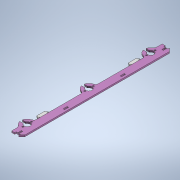
# Autodesk Inventor part: chassis_1_1-02
Saved by Autodesk Inventor 2022 (Build 260153000, 153)
## iProperties
Created: 2023-03-24
Part Number: chassis_1_1-02
Material: 一般
Document SubType Name: Modeling
Designer: Johnny Jou
Density: 1 g/cm^3
Appearance: 預設
Author: Johnny Jou
Autodesk Inventor part; units mm, degrees
ref_plane "YZ Plane" through (0, 0, 0) normal (1, 0, 0) x (0, 1, 0)
ref_plane "XZ Plane" through (0, 0, 0) normal (0, 1, 0) x (-1, 0, 0)
ref_plane "XY Plane" through (0, 0, 0) normal (0, 0, 1) x (1, 0, 0)
sketch "草圖1" plane through (0, 0, 0) normal (0, 1, 0) x (-1, 0, 0)
  line L0 (0, 0) -> (0, -296)
  arc A0 (15, -160.4599) -> (15, -135.5401) centre (16, -148) ccw
  circle A1 centre (16, -148) radius 26 construction
  line L1 (15, -286) -> (15, -160.4599)
  line L2 (15, -135.5401) -> (15, -10)
  circle A2 centre (16, -139.5) radius 1.5
  circle A3 centre (16, -156.5) radius 1.5
  line L3 (20, 0) -> (20, -10)
  line L4 (20, -10) -> (15, -10)
  line L5 (0, -10) -> (0, 0)
  line L6 (6, 0) -> (6, -3)
  line L7 (6, -3) -> (14, -3)
  line L8 (14, -3) -> (14, 0)
  line L9 (0, 0) -> (6, 0)
  line L10 (14, 0) -> (20, 0)
  line L11 (15, 0) -> (14, 0)
  line L12 (6, 0) -> (0, 0)
  line L13 (20, -296) -> (20, -286)
  line L14 (20, -286) -> (15, -286)
  line L15 (0, -290) -> (0, -296)
  line L16 (6, -296) -> (6, -293)
  line L17 (6, -293) -> (14, -293)
  line L18 (14, -293) -> (14, -296)
  line L19 (0, -296) -> (6, -296)
  line L20 (14, -296) -> (20, -296)
  dimension "d1" = 15
  dimension "d2" = 25
  dimension "d3" = 52
  dimension "d4" = 16
  dimension "d6" = 3
  dimension "d7" = 17
  dimension "d8" = 8.5
  dimension "d9" = 10
  dimension "d10" = 20
  dimension "d11" = 8
  dimension "d12" = 3
  dimension "d13" = 6
  dimension "d15" = 3
  dimension "d16" = 8
  dimension "d17" = 6
  dimension "d34" = 296
  dimension "d35" = 148
  dimension "d36" = 10
  dimension "d55" = 8.5
  dimension "d56" = 15
  dimension "d57" = 15
  constraints: 42 end point, 10 parallel, 6 horizontal, 6 perpendicular, 4 centre point, 2 coincident, 2 collinear, 2 point on circle, 1 equal radius, 1 vertical alignment
  measures "d1" distance of L11.start L0.start
  measures "d2" diameter of A0
  measures "d3" diameter of A1
  measures "d4" distance from line of L0 A0.centre
  measures "d6" diameter of A2
  measures "d7" distance of A3.centre A2.centre
  measures "d8" distance of A0.centre A3.centre
  measures "d9" distance of L3.start L3.end
  measures "d10" distance between parallel lines of L0 L3
  measures "d11" distance of L6.end L7.end
  measures "d12" distance of L7.end L8.end
  measures "d13" distance between parallel lines of L5 L6
  measures "d15" distance of L17.end L18.end
  measures "d16" distance of L16.end L17.end
  measures "d17" distance between parallel lines of L0 L16
  measures "d34" distance of L0.start L0.end
  measures "d35" distance from line of L19 A0.centre
  measures "d36" distance of L13.start L13.end
  measures "d55" distance of A0.centre A2.centre
  measures "d56" distance between parallel lines of L0 L1
  measures "d57" distance between parallel lines of L0 L2
extrude "擠出1" add sketch "草圖1" along normal blind 3
sketch "草圖2" plane through (0, 3, 0) normal (0, 1, 0) x (1, 0, 0)
  line L0 (-7, 200) -> (-4, 200)
  line L1 (-4, 200) -> (-4, 208)
  line L2 (-4, 208) -> (-7, 208)
  line L3 (-7, 208) -> (-7, 200)
  arc A0 (-15, 160.4599) -> (-15, 135.5401) centre (-16, 148) ccw projected
  line L4 (-15, 135.5401) -> (-15, 10) projected
  circle A1 centre (-16, 148) radius 12.5 construction
  line L5 (0, 0) -> (0, 296) projected
  line L6 (-11, 4) -> (-8, 4)
  line L7 (-8, 4) -> (-8, 10)
  line L8 (-8, 10) -> (-11, 10)
  line L9 (-11, 10) -> (-11, 4)
  line L10 (-14, 3) -> (-6, 3) projected
  line L11 (-11, 286) -> (-8, 286)
  line L12 (-8, 286) -> (-8, 292)
  line L13 (-8, 292) -> (-11, 292)
  line L14 (-11, 292) -> (-11, 286)
  line L15 (-6, 293) -> (-14, 293) projected
  line L16 (-7, 88) -> (-4, 88)
  line L17 (-4, 88) -> (-4, 96)
  line L18 (-4, 96) -> (-7, 96)
  line L19 (-7, 96) -> (-7, 88)
  line L20 (-15, 286) -> (-15, 160.4599) projected
  dimension "d20" = 8
  dimension "d21" = 3
  dimension "d22" = 60
  dimension "d23" = 4
  dimension "d24" = 6
  dimension "d25" = 3
  dimension "d27" = 1
  dimension "d28" = 6
  dimension "d29" = 3
  dimension "d31" = 1
  dimension "d58" = 3
  dimension "d59" = 8
  dimension "d60" = 60
  dimension "d69" = 4
  dimension "d70" = 4
  constraints: 32 end point, 8 parallel, 4 horizontal, 4 perpendicular, 1 coincident, 1 collinear, 3 other
  measures "d20" distance of L2.end L0.start
  measures "d21" distance of L1.end L2.end
  measures "d22" distance from line of A0.centre L2
  measures "d23" distance between parallel lines of L5 L1
  measures "d24" distance of L8.end L6.start
  measures "d25" distance of L7.end L8.end
  measures "d27" distance between parallel lines of L10 L6
  measures "d28" distance of L13.end L11.start
  measures "d29" distance of L11.start L11.end
  measures "d31" distance between parallel lines of L15 L13
  measures "d58" distance of L17.end L18.end
  measures "d59" distance of L16.end L17.end
  measures "d60" distance from line of A0.centre L16
  measures "d69" distance between parallel lines of L20 L14
  measures "d70" distance between parallel lines of L4 L9
extrude "擠出2" cut sketch "草圖2" against normal up to surface (3 mm away)
sketch "草圖3" plane through (0, 3, 0) normal (0, 1, 0) x (1, 0, 0)
  arc A0 (-15, 160.4599) -> (-15, 135.5401) centre (-16, 148) ccw projected
  circle A1 centre (-16, 148) radius 6
  point P0 (0, 0)
  dimension "d37" = 12
  constraints: 1 centre point, 1 coincident
  measures "d37" diameter of A1
extrude "擠出3" cut sketch "草圖3" against normal up to surface (3 mm away)
sketch "草圖4" plane through (0, 3, 0) normal (0, 1, 0) x (1, 0, 0)
  circle A0 centre (-16, 148) radius 6 projected
  arc A1 (-15, 160.4599) -> (-15, 135.5401) centre (-16, 148) ccw projected
  circle A2 centre (-16, 139.5) radius 1.5 projected
  circle A3 centre (-16, 156.5) radius 1.5 projected
  circle A4 centre (-16, 26.5) radius 12.5
  circle A5 centre (-16, 26.5) radius 6
  circle A6 centre (-16, 35) radius 1.5
  circle A7 centre (-16, 18) radius 1.5
  line L0 (-15, 135.5401) -> (-15, 10) projected
  circle A8 centre (-16, 269.5) radius 12.5
  circle A9 centre (-16, 269.5) radius 6
  circle A10 centre (-16, 278) radius 1.5
  circle A11 centre (-16, 261) radius 1.5
  point P0 (0, 0)
  point P1 (-15, 14.0401)
  point P2 (-15, 38.9599)
  dimension "d40" = 3
  dimension "d41" = 12
  dimension "d42" = 25
  dimension "d43" = 17
  dimension "d44" = 8.5
  dimension "d45" = 121.5
  dimension "d48" = 243
  constraints: 8 centre point, 3 vertical alignment, 2 coincident, 1 equal radius, 1 vertical, 8 other
  measures "d40" diameter of A6
  measures "d41" diameter of A5
  measures "d42" diameter of A4
  measures "d43" distance of A7.centre A6.centre
  measures "d44" distance of A4.centre A6.centre
  measures "d45" distance of A0.centre A4.centre
  measures "d48" distance of A4.centre A8.centre
extrude "擠出4" add sketch "草圖4" against normal up to surface (3 mm away) contours A4 L0 A7 A5 A6 | L0 A6 A5 A7 A4 | A8
sketch "草圖6" plane through (0, 3, 0) normal (0, 1, 0) x (1, 0, 0)
  arc A0 (-15, 32.4161) -> (-15, 20.5839) centre (-16, 26.5) ccw projected
  arc A1 (-15, 275.4161) -> (-15, 263.5839) centre (-16, 269.5) ccw projected
  line L0 (-15, 275.4161) -> (-15, 263.5839) projected
  circle A2 centre (-16, 269.5) radius 6
  line L1 (-15, 32.4161) -> (-15, 20.5839) projected
  circle A3 centre (-16, 26.5) radius 6
  point P0 (0, 0)
  point P1 (-15, 263.5839)
  point P2 (-15, 32.4161)
  constraints: 2 coincident, 6 other
extrude "擠出" cut sketch "草圖6" against normal up to surface (3 mm away) contours A3 L1 | L0 A1 | A2 L0
chamfer "倒角1" distance 6 angle 45 1 edges at (0, 1.5, -296)
chamfer "倒角2" distance 6 angle 45 1 edges at (0, 1.5, 0)
sketch "草圖8" plane through (0, 3, 0) normal (0, 1, 0) x (1, 0, 0)
  circle A0 centre (-16, 269.5) radius 6 projected
  circle A1 centre (-16, 26.5) radius 6 projected
  line L0 (-15, 262.118) -> (-15, 259.882) projected
  arc A2 (-15, 262.118) -> (-15, 259.882) centre (-16, 261) ccw projected
  line L1 (0, 6) -> (-6, 0) projected
  line L2 (0, 6) -> (0, 290) projected
  line L3 (-6, 296) -> (0, 290) projected
  line L4 (-6, 296) -> (-6, 293) projected
  line L5 (-6, 293) -> (-14, 293) projected
  line L6 (-14, 293) -> (-14, 296) projected
  line L7 (-14, 296) -> (-20, 296) projected
  line L8 (-20, 296) -> (-20, 286) projected
  line L9 (-20, 286) -> (-15, 286) projected
  line L10 (-15, 286) -> (-15, 281.9599) projected
  arc A3 (-15, 281.9599) -> (-15, 257.0401) centre (-16, 269.5) ccw projected
  line L11 (-15, 257.0401) -> (-15, 160.4599) projected
  arc A4 (-15, 160.4599) -> (-15, 135.5401) centre (-16, 148) ccw projected
  line L12 (-15, 135.5401) -> (-15, 38.9599) projected
  arc A5 (-15, 38.9599) -> (-15, 14.0401) centre (-16, 26.5) ccw projected
  line L13 (-20, 10) -> (-20, 0) projected
  line L14 (-20, 0) -> (-14, 0) projected
  line L15 (-14, 0) -> (-14, 3) projected
  line L16 (-14, 3) -> (-6, 3) projected
  line L17 (-6, 3) -> (-6, 0) projected
  arc A6 (-15, 36.118) -> (-15, 33.882) centre (-16, 35) ccw projected
  line L18 (-15, 36.118) -> (-15, 33.882) projected
  circle A7 centre (-16, 148) radius 6 projected
  line L19 (-4, 208) -> (-4, 200) projected
  line L20 (-4, 200) -> (-7, 200) projected
  line L21 (-7, 200) -> (-7, 208) projected
  line L22 (-7, 208) -> (-4, 208) projected
  line L23 (-4, 88) -> (-7, 88) projected
  line L24 (-7, 88) -> (-7, 96) projected
  line L25 (-7, 96) -> (-4, 96) projected
  line L26 (-4, 96) -> (-4, 88) projected
  line L27 (-8, 292) -> (-8, 286) projected
  line L28 (-8, 286) -> (-11, 286) projected
  line L29 (-11, 286) -> (-11, 292) projected
  line L30 (-11, 292) -> (-8, 292) projected
  line L31 (-8, 4) -> (-11, 4) projected
  line L32 (-11, 4) -> (-11, 10) projected
  line L33 (-8, 10) -> (-8, 4) projected
  circle A8 centre (-16, 139.5) radius 1.5 projected
  circle A9 centre (-16, 156.5) radius 1.5 projected
  arc A10 (-15, 279.118) -> (-15, 276.882) centre (-16, 278) ccw projected
  line L34 (-15, 279.118) -> (-15, 276.882) projected
  circle A11 centre (-20, 43.5367) radius 5
  line L35 (-15, 135.5401) -> (-15, 38.9599) projected
  circle A12 centre (-27.7647, 10) radius 7.7647
  circle A13 centre (-20, 130.9633) radius 5
  circle A14 centre (-20, 165.0367) radius 5
  circle A15 centre (-20, 252.4633) radius 5
  arc A16 (-15, 38.9599) -> (-20, 9.6573) centre (-16, 26.5) ccw projected
  line L36 (-20, 9.6573) -> (-20, 0) projected
  arc A17 (-15, 160.4599) -> (-15, 135.5401) centre (-16, 148) ccw projected
  line L37 (-15, 257.0401) -> (-15, 160.4599) projected
  circle A18 centre (-27.7647, 286) radius 7.7647
  line L38 (-20, 296) -> (-20, 286) projected
  line L39 (-11, 10) -> (-8, 10) projected
  line L40 (-15, 14.0401) -> (-15, 10) projected
  line L41 (-15, 10) -> (-20, 10) projected
  point P0 (0, 0)
  point P1 (-23.2569, 279.6778)
  point P2 (-18.8571, 257.3309)
  point P3 (-15, 252.4633)
  point P4 (-15, 165.0367)
  point P5 (-18.8571, 160.1691)
  point P6 (-18.8571, 135.8309)
  point P7 (-15, 130.9633)
  point P8 (-15, 43.5367)
  point P9 (-18.8571, 38.6691)
  point P10 (-23.2569, 16.3222)
  point P11 (-20, 4.6573)
  point P12 (-27.9283, 17.763)
  dimension "d71" = 10
  constraints: 8 tangent, 4 centre point, 3 equal radius, 2 vertical, 8 other
  measures "d71" diameter of A11
extrude "擠出6" add sketch "草圖8" against normal up to surface (3 mm away) contours A12 A5 L40 L41 | L9 L10 A3 A18 | A3 L11 A15 | A11 L12 A5 | L11 A4 A14 | A13 A4 L12
sketch "草圖9" plane through (0, 3, 0) normal (0, 1, 0) x (1, 0, 0)
  circle A0 centre (-16, 269.5) radius 6 projected
  circle A1 centre (-16, 26.5) radius 6 projected
  line L0 (-15, 262.118) -> (-15, 259.882) projected
  arc A2 (-15, 262.118) -> (-15, 259.882) centre (-16, 261) ccw projected
  line L1 (0, 6) -> (-6, 0) projected
  line L2 (0, 6) -> (0, 290) projected
  line L3 (-6, 296) -> (0, 290) projected
  line L4 (-6, 296) -> (-6, 293) projected
  line L5 (-6, 293) -> (-14, 293) projected
  line L6 (-14, 293) -> (-14, 296) projected
  line L7 (-14, 296) -> (-20, 296) projected
  line L8 (-20, 296) -> (-20, 286) projected
  arc A3 (-23.2569, 279.6778) -> (-20, 286) centre (-27.7647, 286) ccw projected
  arc A4 (-23.2569, 279.6778) -> (-18.8571, 257.3309) centre (-16, 269.5) ccw projected
  arc A5 (-15, 252.4633) -> (-18.8571, 257.3309) centre (-20, 252.4633) ccw projected
  line L9 (-15, 252.4633) -> (-15, 165.0367) projected
  arc A6 (-18.8571, 160.1691) -> (-15, 165.0367) centre (-20, 165.0367) ccw projected
  arc A7 (-18.8571, 160.1691) -> (-18.8571, 135.8309) centre (-16, 148) ccw projected
  arc A8 (-15, 130.9633) -> (-18.8571, 135.8309) centre (-20, 130.9633) ccw projected
  line L10 (-15, 130.9633) -> (-15, 43.5367) projected
  arc A9 (-18.8571, 38.6691) -> (-15, 43.5367) centre (-20, 43.5367) ccw projected
  arc A10 (-18.8571, 38.6691) -> (-23.2569, 16.3222) centre (-16, 26.5) ccw projected
  arc A11 (-20, 10) -> (-23.2569, 16.3222) centre (-27.7647, 10) ccw projected
  line L11 (-20, 10) -> (-20, 0) projected
  line L12 (-20, 0) -> (-14, 0) projected
  line L13 (-14, 0) -> (-14, 3) projected
  line L14 (-14, 3) -> (-6, 3) projected
  line L15 (-6, 3) -> (-6, 0) projected
  arc A12 (-15, 36.118) -> (-15, 33.882) centre (-16, 35) ccw projected
  line L16 (-15, 36.118) -> (-15, 33.882) projected
  circle A13 centre (-16, 148) radius 6 projected
  line L17 (-4, 208) -> (-4, 200) projected
  line L18 (-4, 200) -> (-7, 200) projected
  line L19 (-7, 200) -> (-7, 208) projected
  line L20 (-7, 208) -> (-4, 208) projected
  line L21 (-4, 88) -> (-7, 88) projected
  line L22 (-7, 88) -> (-7, 96) projected
  line L23 (-7, 96) -> (-4, 96) projected
  line L24 (-4, 96) -> (-4, 88) projected
  line L25 (-8, 292) -> (-8, 286) projected
  line L26 (-8, 286) -> (-11, 286) projected
  line L27 (-11, 286) -> (-11, 292) projected
  line L28 (-11, 292) -> (-8, 292) projected
  line L29 (-8, 4) -> (-11, 4) projected
  line L30 (-11, 4) -> (-11, 10) projected
  line L31 (-8, 10) -> (-8, 4) projected
  circle A14 centre (-16, 139.5) radius 1.5 projected
  circle A15 centre (-16, 156.5) radius 1.5 projected
  arc A16 (-15, 279.118) -> (-15, 276.882) centre (-16, 278) ccw projected
  line L32 (-15, 279.118) -> (-15, 276.882) projected
  arc A17 (-15, 19.118) -> (-15, 16.882) centre (-16, 18) ccw projected
  circle A18 centre (-16, 18) radius 1.5
  line L33 (-15, 36.118) -> (-15, 33.882) projected
  circle A19 centre (-16, 35) radius 1.5
  circle A20 centre (-16, 261) radius 1.5
  circle A21 centre (-16, 278) radius 1.5
  line L34 (-28.5, 267) -> (-21.4544, 267)
  line L35 (-21.4544, 267) -> (-21.4544, 272)
  line L36 (-21.4544, 272) -> (-28.5, 272)
  line L37 (-28.5, 272) -> (-28.5, 267)
  circle A22 centre (-16, 269.5) radius 6 projected
  arc A23 (-23.2569, 279.6778) -> (-18.8571, 257.3309) centre (-16, 269.5) ccw projected
  line L38 (-28.5, 145.5) -> (-21.4544, 145.5)
  line L39 (-21.4544, 145.5) -> (-21.4544, 150.5)
  line L40 (-21.4544, 150.5) -> (-28.5, 150.5)
  line L41 (-28.5, 150.5) -> (-28.5, 145.5)
  circle A24 centre (-16, 148) radius 6 projected
  line L42 (-28.5, 24) -> (-21.4544, 24)
  line L43 (-21.4544, 24) -> (-21.4544, 29)
  line L44 (-21.4544, 29) -> (-28.5, 29)
  line L45 (-28.5, 29) -> (-28.5, 24)
  arc A25 (-18.8571, 38.6691) -> (-23.2569, 16.3222) centre (-16, 26.5) ccw projected
  circle A26 centre (-16, 26.5) radius 6 projected
  line L46 (-11, 10) -> (-8, 10) projected
  line L47 (-15, 19.118) -> (-15, 16.882) projected
  arc A27 (-15, 19.118) -> (-15, 16.882) centre (-16, 18) ccw projected
  point P0 (0, 0)
  point P1 (-28.2474, 272)
  point P2 (-28.2474, 267)
  point P3 (-28.2474, 150.5)
  point P4 (-28.2474, 145.5)
  point P5 (-28.2474, 29)
  point P6 (-28.2474, 24)
  point P7 (-15, 33.882)
  point P8 (-21.8029, 14.9747)
  point P9 (-20.38, 12.3993)
  point P10 (-21.4544, 19)
  point P11 (-21.4544, 14.5244)
  dimension "d74" = 5
  dimension "d75" = 5
  dimension "d76" = 5
  constraints: 24 end point, 6 parallel, 4 coincident, 3 horizontal, 3 perpendicular, 3 tangent, 2 point on circle, 20 other
  measures "d74" distance of L36.end L34.start
  measures "d75" distance of L40.end L38.start
  measures "d76" distance of L44.end L42.start
extrude "擠出7" cut sketch "草圖9" against normal up to surface (3 mm away) contours A0 L34 A4 L36 | L40 A13 L38 A7 | L44 A1 L42 A10 | A10 L45 L44 | A10 L42 L45 | A20 L0 | A19 L16 | A21 L32 | L47 A17 | A18 L47
fillet "圓角1" radius 0.5 12 edges at (-21.4544, 1.5, -272) (-28.2474, 1.5, -272) (-21.4544, 1.5, -267) (-28.2474, 1.5, -267) (-21.4544, 1.5, -145.5) (-28.2474, 1.5, -145.5) (-21.4544, 1.5, -150.5) (-28.2474, 1.5, -150.5) (-21.4544, 1.5, -29) (-28.2474, 1.5, -29) (-28.2474, 1.5, -24) (-21.4544, 1.5, -24)
sketch "草圖11" plane through (0, 3, 0) normal (0, 1, 0) x (1, 0, 0)
  line L0 (-15, 130.9633) -> (-15, 43.5367) projected
  line L1 (-15, 252.4633) -> (-15, 165.0367) projected
  line L2 (-16, 245.5) -> (-15, 245.5)
  line L3 (-16, 248.5) -> (-16, 245.5)
  line L4 (-21, 245.5) -> (-16, 248.5)
  line L5 (-15, 230.5) -> (-16, 230.5)
  line L6 (-16, 230.5) -> (-16, 227.5)
  line L7 (-21, 230.5) -> (-21, 245.5)
  line L8 (-16, 227.5) -> (-21, 230.5)
  arc A0 (-21.3227, 266.7308) -> (-21.3227, 272.2692) centre (-16, 269.5) ccw projected
  arc A1 (-21.3227, 145.2308) -> (-21.3227, 150.7692) centre (-16, 148) ccw projected
  line L9 (-16, 148) -> (0, 148)
  line L10 (-16, 50.5) -> (-15, 50.5)
  line L11 (-16, 47.5) -> (-16, 50.5)
  line L12 (-21, 50.5) -> (-16, 47.5)
  line L13 (-15, 65.5) -> (-16, 65.5)
  line L14 (-16, 65.5) -> (-16, 68.5)
  line L15 (-21, 65.5) -> (-21, 50.5)
  line L16 (-16, 68.5) -> (-21, 65.5)
  point P0 (0, 0)
  dimension "d80" = 15
  dimension "d81" = 3
  dimension "d82" = 1
  dimension "d83" = 3
  dimension "d84" = 1
  dimension "d85" = 24
  constraints: 30 end point, 8 symmetric about line, 3 horizontal, 3 vertical, 2 horizontal alignment, 2 point on line
  measures "d80" distance of L7.start L4.start
  measures "d81" distance of L5.end L6.end
  measures "d82" distance of L5.start L5.end
  measures "d83" distance of L3.start L2.start
  measures "d84" distance of L2.start L2.end
  measures "d85" distance from line of A0.centre L2
extrude "擠出8" add sketch "草圖11" against normal up to surface (3 mm away) separate body
equation "\"d8\" = 0.5 * d7"
equation "\"d35\" = 0.5 * d34"
equation "\"d31\" = d27"
equation "\"d58\" = d21"
equation "\"d59\" = d20"
equation "\"d60\" = d22"
equation "\"d44\" = 0.5 * d43"
equation "\"d48\" = 2 * d45"
